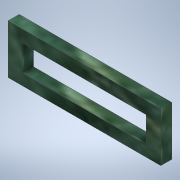
# Autodesk Inventor part: lcd1
Saved by Autodesk Inventor 2021 (Build 250183000, 183)
## iProperties
Created: 2021-07-13
Part Number: lcd1
Material: Generic
Document SubType Name: Modeling
Designer: Dell
Density: 1 g/cm^3
Appearance: Default
Author: Dell
Autodesk Inventor part; units mm, degrees
ref_plane "YZ Plane" through (0, 0, 0) normal (1, 0, 0) x (0, 1, 0)
ref_plane "XZ Plane" through (0, 0, 0) normal (0, 1, 0) x (-1, 0, 0)
ref_plane "XY Plane" through (0, 0, 0) normal (0, 0, 1) x (1, 0, 0)
sketch "Sketch1" plane through (0, 0, 0) normal (0, 0, 1) x (1, 0, 0)
  line L0 (0, 11.9936) -> (13.6628, 11.9936)
  line L1 (13.6628, 11.9936) -> (13.6628, 7.6017)
  line L2 (13.6628, 7.6017) -> (0, 7.6017)
  line L3 (0, 7.6017) -> (0, 11.9936)
  line L4 (1.2716, 10.8956) -> (12.3453, 10.8956)
  line L5 (12.3453, 10.8956) -> (12.3453, 8.5742)
  line L6 (12.3453, 8.5742) -> (1.2716, 8.5742)
  line L7 (1.2716, 8.5742) -> (1.2716, 10.8956)
  point P0 (0, 0)
  constraints: 16 end point, 4 parallel, 2 horizontal, 2 perpendicular
extrude "Extrusion1" add sketch "Sketch1" along normal blind 1
body "Solid1"
